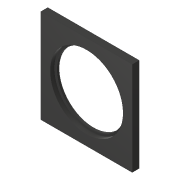
# Autodesk Inventor part: sphericalLensHolder
Saved by Autodesk Inventor 2018 (Build 220112000, 112)
## iProperties
Created: 2017-03-28
Part Number: sphericalLensHolder
Material: ABS Plastic
Document SubType Name: Modeling
Designer: sawaiz
Density: 1.06 g/cm^3
Appearance: Smooth - Black
Author: sawaiz
Autodesk Inventor part; units mm, degrees
ref_plane "YZ Plane" through (0, 0, 0) normal (1, 0, 0) x (0, 1, 0)
ref_plane "XZ Plane" through (0, 0, 0) normal (0, 1, 0) x (-1, 0, 0)
ref_plane "XY Plane" through (0, 0, 0) normal (0, 0, 1) x (1, 0, 0)
sketch "Sketch1" plane through (0, 0, 0) normal (0, 0, 1) x (1, 0, 0)
  line L0 (-63.3984, -65.0875) -> (63.3984, -65.0875)
  line L1 (63.3984, -65.0875) -> (63.3984, 65.0875)
  line L2 (63.3984, 65.0875) -> (-63.3984, 65.0875)
  line L3 (-63.3984, 65.0875) -> (-63.3984, -65.0875)
  line L4 (-63.3984, -65.0875) -> (63.3984, 65.0875) construction
  line L5 (63.3984, -65.0875) -> (-63.3984, 65.0875) construction
  point P0 (0, 0)
  dimension "d0" = 126.7968
  dimension "d1" = 130.175
  constraints: 12 end point, 2 midpoint, 2 parallel, 1 horizontal, 1 perpendicular
  measures "d0" distance of L1.end L2.end
  measures "d1" distance of L0.end L1.end
extrude "Extrusion1" add sketch "Sketch1" along normal blind 9.525
sketch "Sketch2" plane through (0, 0, 9.525) normal (0, 0, 1) x (1, 0, 0)
  circle A0 centre (0, 0) radius 50.8508
  dimension "d4" = 101.7016
  constraints: 1 centre point, 1 coincident
  measures "d4" diameter of A0
extrude "Extrusion2" cut sketch "Sketch2" against normal blind 6.35
sketch "Sketch3" plane through (0, 0, 3.175) normal (0, 0, 1) x (1, 0, 0)
  circle A0 centre (0, 0) radius 47.625
  dimension "d7" = 95.25
  constraints: 1 centre point, 1 coincident
  measures "d7" diameter of A0
extrude "Extrusion3" cut sketch "Sketch3" along normal through all both and the other way through all
equation "\"d0\" = width - 2 * alignmentGrooveClearance"
equation "\"d1\" = height + 2 * alignmentGrooveDepth"
equation "\"d2\" = lensMountThickness"
equation "\"d4\" = lensDiameter + alignmentGrooveClearance"
equation "\"d5\" = lensInsetDepth"
equation "\"d7\" = lensDiameter - lensInsetDepth"
equation "\"d8\" = lensInsetDepth"
equation "\"caseThickness\" = 6.35"
equation "\"alignmentGrooveDepth\" = 1.5875"
equation "\"alignmentGrooveClearance\" = 0.1016"
equation "\"aerogelHolderDepth\" = 38.24501"
equation "\"height\" = 127"
equation "\"width\" = 127"
equation "\"depth\" = 247.57228"
equation "\"mirrorAngle\" = 2.5deg"
equation "\"mirrorThickness\" = 3.175"
equation "\"fresnelThickness\" = 0.254"
equation "\"focalLength\" = 185.82488"
equation "\"ior\" = 1.49"
equation "\"centerThickness\" = 1.27"
equation "\"fresnelAngle\" = 90deg"
equation "\"fresnelEffectiveDiameter\" = 152.4"
equation "\"fresnelGrooveWidth\" = 9.525"
equation "\"frontPanelThickness\" = 1.5875"
equation "\"lensMountThickness\" = 9.525"
equation "\"lensInsetDepth\" = 6.35"
equation "\"lensDiameter\" = 101.6"
equation "\"lensCenterThickness\" = 16.99999"
body "Solid1"
